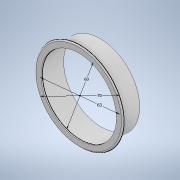
# Autodesk Inventor part: Hole64mm
Saved by Autodesk Inventor 2022 (Build 260153000, 153)
## iProperties
Created: 2021-12-15
Part Number: Hole64mm
Material: Generic
Document SubType Name: Modeling
Designer: dangl
Density: 1 g/cm^3
Appearance: Default
Author: dangl
Autodesk Inventor part; units mm, degrees
ref_plane "YZ Plane" through (0, 0, 0) normal (1, 0, 0) x (0, 1, 0)
ref_plane "XZ Plane" through (0, 0, 0) normal (0, 1, 0) x (-1, 0, 0)
ref_plane "XY Plane" through (0, 0, 0) normal (0, 0, 1) x (1, 0, 0)
sketch "Sketch1" plane through (0, 0, 0) normal (0, 0, 1) x (1, 0, 0)
  circle A0 centre (0, 0) radius 31.5
  circle A1 centre (0, 0) radius 30
  circle A2 centre (0, 0) radius 35
  dimension "d0" = 63
  dimension "d1" = 60
  dimension "d2" = 70
  constraints: 3 centre point, 3 coincident
  measures "d0" diameter of A0
  measures "d1" diameter of A1
  measures "d2" diameter of A2
extrude "Extrusion1" add sketch "Sketch1" along normal blind 1 contours A0 | A2
extrude "Extrusion2" add sketch "Sketch1" against normal blind 17 contours A0
fillet "Fillet1" radius 1 1 edges at (-35, 0, 1)
fillet "Fillet2" radius 1 1 edges at (-31.5, 0, -17)
body "Solid1"
